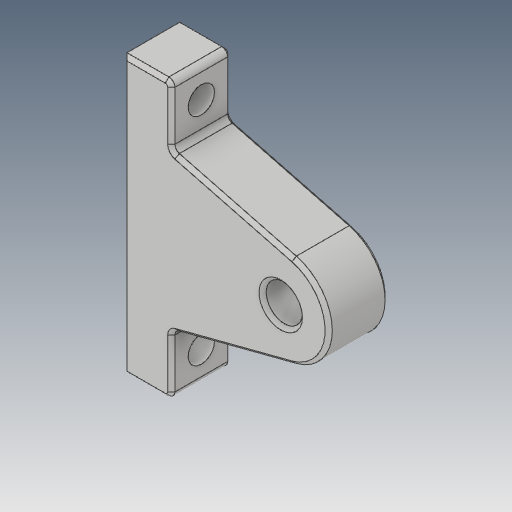
# Autodesk Inventor part: hinge-axis_mount
Saved by Autodesk Inventor 2018 (Build 220112000, 112)
## iProperties
Created: 2019-03-07
Part Number: hinge-axis_mount
Material: Generic
Document SubType Name: Modeling
Designer: Tsche
Density: 1 g/cm^3
Appearance: Default
Author: Tsche
Autodesk Inventor part; units mm, degrees
ref_plane "YZ Plane" through (0, 0, 0) normal (1, 0, 0) x (0, 1, 0)
ref_plane "XZ Plane" through (0, 0, 0) normal (0, 1, 0) x (-1, 0, 0)
ref_plane "XY Plane" through (0, 0, 0) normal (0, 0, 1) x (1, 0, 0)
sketch "Sketch1" plane through (0, 0, 0) normal (0, 0, 1) x (1, 0, 0)
  line L0 (0, 0) -> (0, 11.5)
  line L1 (0, 11.5) -> (4, 11.5)
  line L2 (4, 11.5) -> (4, 6.5)
  line L3 (4, 6.5) -> (14.1296, 3.8718)
  line L4 (-3.5573, 0) -> (21.3437, 0) construction
  circle A0 centre (13.125, 0) radius 1.5125
  arc A1 (17.125, 0) -> (14.1296, 3.8718) centre (13.125, 0) ccw
  line L5 (0, 0) -> (0, -11.5)
  line L6 (0, -11.5) -> (4, -11.5)
  line L7 (4, -11.5) -> (4, -6.5)
  line L8 (4, -6.5) -> (14.1296, -3.8718)
  arc A2 (14.1296, -3.8718) -> (17.125, 0) centre (13.125, 0) ccw
  dimension "d0" = 3.025
  dimension "d1" = 13.125
  dimension "d2" = 4
  dimension "d3" = 11.5
  dimension "d4" = 4
  dimension "d5" = 5
  constraints: 16 end point, 4 point on circle, 4 symmetric about line, 3 centre point, 2 perpendicular, 2 point on line, 1 concentric, 1 tangent, 1 vertical, 1 other
  measures "d0" diameter of A0
  measures "d1" distance from line of A0.centre L0
  measures "d2" radius of A1
  measures "d3" distance between parallel lines of L1 L4
  measures "d4" distance of L0.end L1.end
  measures "d5" distance of L1.end L2.end
extrude "Extrusion1" add sketch "Sketch1" along normal blind 5
fillet "Fillet1" radius 0.5 4 edges at (4, 6.5, 2.5) (4, -6.5, 2.5) (4, -11.5, 2.5) (4, 11.5, 2.5)
chamfer "Chamfer1" distance 0.3 angle 45 26 edges at (16.2887, 2.4476, 0) (9.252, -5.1373, 0) (4.1045, -6.5809, 0) (4, -8.9434, 0) (3.8536, -11.3536, 0) (1.75, -11.5, 0) (9.252, 5.1373, 0) (4.1045, 6.5809, 0) (4, 8.9434, 0) (3.8536, 11.3536, 0) (1.75, 11.5, 0) (11.6125, 0, 0) (0, 5.75, 0) (4, -8.9434, 5) (4.1045, -6.5809, 5) (9.252, -5.1373, 5) (16.2887, 2.4476, 5) (9.252, 5.1373, 5) (4.1045, 6.5809, 5) (4, 8.9434, 5) (3.8536, 11.3536, 5) (1.75, 11.5, 5) (3.8536, -11.3536, 5) (1.75, -11.5, 5) (11.6125, 0, 5) (0, -5.75, 5)
hole "Hole1" at (4, 9, 2.5) direction (-1, 0, 0) diameter 2.2 end through all
mirror "Mirror1" about plane through (0, 0, 0) normal (0, 1, 0) of "Hole1"
equation "\"d0\" = bore_clearance"
equation "\"d1\" = -0.5 * finger_width + 0.5 * dist_hinge_points"
equation "\"d9\" = champfer"
equation "\"finger_width\" = 25"
equation "\"finger_thickness\" = 8"
equation "\"finger_part_A_length\" = 42.8625"
equation "\"finger_part_B_length\" = 28.575"
equation "\"finger_link_width\" = 3.5"
equation "\"finger_link_clearence\" = 0.075"
equation "\"tol\" = 0.5 * finger_link_clearence"
equation "\"link_tol\" = 0.254"
equation "\"bore_press\" = 2.925"
equation "\"bore_clearance\" = 3.025"
equation "\"bar_diameter\" = 6.5"
equation "\"bar_thickness\" = 4"
equation "\"bar_width\" = 7"
equation "\"hinge_dist_sym_plane\" = 4"
equation "\"hinge_thickness\" = 3"
equation "\"hinge_act_length_c\" = 7.62"
equation "\"hinge_act_length_bc\" = 16.66875"
equation "\"hinge_act_length_ab\" = 11.049"
equation "\"hinge_act_length_a\" = 21.43125"
equation "\"hinge_guid_length_c\" = 9.525"
equation "\"hinge_guid_length_bc\" = 9.525"
equation "\"hinge_guid_length_ab\" = 17.145"
equation "\"hinge_guid_length_a\" = 17.145"
equation "\"bar_length_bc\" = finger_part_B_length"
equation "\"bar_act_length_ab\" = 40.48125"
equation "\"bar_guid_length_ab\" = 43.275"
equation "\"champfer\" = 0.3"
equation "\"fillet\" = 0.4"
equation "\"gear_diameter\" = 14"
equation "\"dist_finger_BC\" = 56.5"
equation "\"hinge_point\" = 15"
equation "\"dist_hinge_points\" = 51.25"
body "Solid1"
